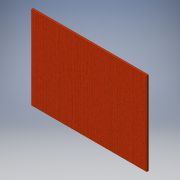
# Autodesk Inventor part: Wine Bottle Rack Back Panel
Saved by Autodesk Inventor 2016 (Build 200138000, 138)
## iProperties
Created: 2017-11-04
Part Number: Wine Bottle Rack Back Panel
Material: Generic
Document SubType Name: Modeling
Designer: mathaetaes
Density: 1 g/cm^3
Appearance: Default
Author: mathaetaes
Autodesk Inventor part; units mm, degrees
ref_plane "YZ Plane" through (0, 0, 0) normal (1, 0, 0) x (0, 1, 0)
ref_plane "XZ Plane" through (0, 0, 0) normal (0, 1, 0) x (-1, 0, 0)
ref_plane "XY Plane" through (0, 0, 0) normal (0, 0, 1) x (1, 0, 0)
sketch "Sketch1" plane through (0, 0, 0) normal (0, 0, 1) x (1, 0, 0)
  line L0 (-138.7249, 170.7086) -> (258.1501, 170.7086)
  line L1 (258.1501, 170.7086) -> (258.1501, -115.0414)
  line L2 (258.1501, -115.0414) -> (-138.7249, -115.0414)
  line L3 (-138.7249, -115.0414) -> (-138.7249, 170.7086)
  point P0 (0, 0)
  dimension "d0" = 396.875
  dimension "d1" = 285.75
  constraints: 8 end point, 2 parallel, 1 horizontal, 1 perpendicular
  measures "d0" distance of L1.end L2.end
  measures "d1" distance of L0.end L1.end
extrude "Board" add sketch "Sketch1" along normal blind 6.35
body "Solid1"
